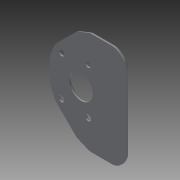
# Autodesk Inventor part: obudowa do czujnikow odleglosci v3,2 - przykrywka
Saved by Autodesk Inventor 2014 (Build 180170000, 170)
## iProperties
Created: 2017-04-19
Part Number: obudowa do czujnikow odleglosci v3,2 - przykrywka
Material: Ogólny
Document SubType Name: Modeling
Designer: hpdc7700
Density: 1 g/cm^3
Appearance: Domyślna
Author: hpdc7700
Autodesk Inventor part; units mm, degrees
ref_plane "YZ Plane" through (0, 0, 0) normal (1, 0, 0) x (0, 1, 0)
ref_plane "XZ Plane" through (0, 0, 0) normal (0, 1, 0) x (-1, 0, 0)
ref_plane "XY Plane" through (0, 0, 0) normal (0, 0, 1) x (1, 0, 0)
sketch "Szkic1" plane through (0, 0, 0) normal (0, 1, 0) x (-1, 0, 0)
  circle A0 centre (20.670805, 15.489913) radius 2.25
  circle A1 centre (20.670805, -15.489913) radius 2.25
  line L0 (-2.43121, 25.942308) -> (-19.284188, 11.800981)
  line L1 (-19.284188, 11.800981) -> (-28.926002, 23.291647)
  line L2 (-28.802745, 24.700479) -> (-28.926002, 23.291647)
  line L3 (-28.802745, 24.700479) -> (-12.715812, 38.199019)
  line L4 (-12.715812, 38.199019) -> (-2.43121, 25.942308)
  line L5 (-26.423342, -11) -> (-26.423342, 11)
  line L6 (-26.423342, 11) -> (-10.423342, 11)
  line L7 (-10.423342, 11) -> (-10.423342, -11)
  line L8 (-10.423342, -11) -> (-26.423342, -11)
  line L9 (-19.284188, -11.800981) -> (-2.43121, -25.942308)
  line L10 (-2.43121, -25.942308) -> (-12.715812, -38.199019)
  line L11 (-12.715812, -38.199019) -> (-28.802745, -24.700479)
  line L12 (-28.926002, -23.291647) -> (-28.802745, -24.700479)
  line L13 (-28.926002, -23.291647) -> (-19.284188, -11.800981)
  arc A2 (24.913446, -19.732553) -> (26.214082, -17.786013) centre (20.670805, -15.489913) ccw
  line L14 (29.391036, -10.116167) -> (26.214082, -17.786013)
  arc A3 (29.391036, -10.116167) -> (30, -7.0547) centre (22, -7.0547) ccw
  line L15 (30, -7.0547) -> (30, 7.0547)
  arc A4 (30, 7.0547) -> (29.391036, 10.116167) centre (22, 7.0547) ccw
  line L16 (26.214082, 17.786013) -> (29.391036, 10.116167)
  arc A5 (26.214082, 17.786013) -> (24.913446, 19.732553) centre (20.670805, 15.489913) ccw
  line L17 (24.913446, 19.732553) -> (9.732553, 34.913446)
  arc A6 (9.732553, 34.913446) -> (7.786013, 36.214082) centre (5.489913, 30.670805) ccw
  line L18 (0.116167, 39.391036) -> (7.786013, 36.214082)
  arc A7 (0.116167, 39.391036) -> (-2.9453, 40) centre (-2.9453, 32) ccw
  line L19 (-2.9453, 40) -> (-18.300026, 40)
  arc A8 (-18.300026, 40) -> (-24.727902, 37.660444) centre (-18.300026, 30) ccw
  line L20 (-24.727902, 37.660444) -> (-26.427876, 36.233997)
  arc A9 (-26.427876, 36.233997) -> (-30, 28.573552) centre (-20, 28.573552) ccw
  line L21 (-30, 28.573552) -> (-30, -28.573552)
  arc A10 (-30, -28.573552) -> (-26.427876, -36.233997) centre (-20, -28.573552) ccw
  line L22 (-26.427876, -36.233997) -> (-24.727902, -37.660444)
  arc A11 (-24.727902, -37.660444) -> (-18.300026, -40) centre (-18.300026, -30) ccw
  line L23 (-18.300026, -40) -> (-2.9453, -40)
  arc A12 (-2.9453, -40) -> (0.116167, -39.391036) centre (-2.9453, -32) ccw
  line L24 (7.786013, -36.214082) -> (0.116167, -39.391036)
  arc A13 (7.786013, -36.214082) -> (9.732553, -34.913446) centre (5.489913, -30.670805) ccw
  line L25 (9.732553, -34.913446) -> (24.913446, -19.732553)
  circle A14 centre (0, -18) radius 2.25
  circle A15 centre (0, 18) radius 2.25
  ellipse E0 centre (5.489913, 0.077944) end of major axis (-3.705883, 0.077944) minor radius 9.366229
  point P0 (0, 0)
  point P1 (0, 0)
  constraints: 52 end point, 24 point on circle, 16 centre point, 1 horizontal, 2 other
extrude "Wyciągnięcie proste1" add sketch "Szkic1" along normal blind 3 contours L0 L1 L2 L3 L4 | L5 L6 L7 L8 | L9 L10 L11 L12 L13 | L25 A13 L24 A12 L23 A11 L22 A10 L21 A9 L20 A8 L19 A7 L18 A6 L17 A5 L16 A4 L15 A3 L14 A2
chamfer "Faza1" distance 2 angle 45 1 edges at (-5.4899, 3, 9.4442)
chamfer "Faza2" distance 2 angle 45 4 edges at (-18.4208, 3, 15.4899) (2.25, 3, 18) (-18.4208, 3, -15.4899) (2.25, 3, -18)
fillet "Zaokrąglenie1" radius 3 24 edges at (30, 3, 0) (29.0631, 3, -32.7997) (25.5779, 3, -36.9472) (21.7202, 3, -39.3969) (10.6227, 3, -40) (1.3846, 3, -39.8463) (-3.9511, 3, -37.8026) (-8.8233, 3, -35.6596) (-17.323, 3, -27.323) (-25.6596, 3, -18.8233) (-27.8026, 3, -13.9511) (-29.8463, 3, -8.6154) (-30, 3, 0) (-29.8463, 3, 8.6154) (-27.8026, 3, 13.9511) (-25.6596, 3, 18.8233) (-17.323, 3, 27.323) (-8.8233, 3, 35.6596) (-3.9511, 3, 37.8026) (1.3846, 3, 39.8463) (10.6227, 3, 40) (21.7202, 3, 39.3969) (25.5779, 3, 36.9472) (29.0631, 3, 32.7997)
